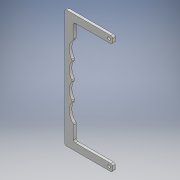
# Autodesk Inventor part: handle_v3
Saved by Autodesk Inventor 2018 (Build 220112000, 112)
## iProperties
Created: 2018-05-21
Part Number: handle_v3
Material: Generic
Document SubType Name: Modeling
Designer: etd
Density: 1 g/cm^3
Appearance: Default
Author: etd
Autodesk Inventor part; units mm, degrees
ref_plane "YZ Plane" through (0, 0, 0) normal (1, 0, 0) x (0, 1, 0)
ref_plane "XZ Plane" through (0, 0, 0) normal (0, 1, 0) x (-1, 0, 0)
ref_plane "XY Plane" through (0, 0, 0) normal (0, 0, 1) x (1, 0, 0)
sketch "Sketch1" plane through (0, 0, 0) normal (0, 1, 0) x (-1, 0, 0)
  line L0 (0, 0) -> (50, 0) construction
  line L1 (0, 0) -> (0, -62.5) construction
  line L2 (0, -62.5) -> (-4, -62.5) construction
  line L3 (40, -58.5) -> (-4, -58.5)
  line L4 (-4, -58.5) -> (-4, -66.5)
  line L5 (-4, -66.5) -> (50, -66.5)
  line L6 (50, -66.5) -> (50, 66.5)
  line L7 (50, 66.5) -> (-4, 66.5)
  line L8 (-4, 66.5) -> (-4, 58.5)
  line L9 (-4, 58.5) -> (40, 58.5)
  line L10 (40, 58.5) -> (40, -58.5)
  point P0 (0, 62.5)
  dimension "d0" = 62.5
  dimension "d1" = 50
  dimension "d2" = 4
  dimension "d3" = 8
  dimension "d4" = 10
  constraints: 22 end point, 5 perpendicular, 4 horizontal, 2 midpoint, 2 vertical, 1 coincident, 1 symmetric about line, 3 other
  measures "d0" distance of L0.start L1.end
  measures "d1" distance of L0.start L0.end
  measures "d2" distance of L1.end L2.end
  measures "d3" distance of L3.end L4.end
  measures "d4" distance between parallel lines of L6 L10
extrude "Plate1" add sketch "Sketch1" along normal blind 3
hole "Hole1" at (0, 0, -62.5) at (0, 0, 62.5) direction (0, 1, 0) diameter 3 end through all
sketch "Sketch2" plane through (0, 3, 0) normal (0, 1, 0) x (1, 0, 0)
  circle A0 centre (0, 62.5) radius 1.5 projected
  circle A1 centre (0, -62.5) radius 1.5 projected
  line L0 (-40, 58.5) -> (-40, -58.5) projected
  line L1 (4, 58.5) -> (-40, 58.5) projected
  line L2 (4, 66.5) -> (4, 58.5) projected
  line L3 (-50, 66.5) -> (4, 66.5) projected
  line L4 (-50, -66.5) -> (-50, 66.5) projected
  line L5 (4, -66.5) -> (-50, -66.5) projected
  line L6 (4, -58.5) -> (4, -66.5) projected
  line L7 (-40, -58.5) -> (4, -58.5) projected
  circle A2 centre (-30, -30) radius 15
  circle A3 centre (-30, -10) radius 15
  circle A4 centre (-30, 10) radius 15
  circle A5 centre (-30, 30) radius 15
  line L8 (-30, 30) -> (-30, -30) construction
  line L9 (-30, 30) -> (-30, 58.5) construction
  line L10 (-30, -30) -> (-30, -58.5) construction
  point P0 (0, 0)
  dimension "d13" = 20
  dimension "d14" = 20
  dimension "d15" = 30
  dimension "d16" = 20
  dimension "d17" = 10
  constraints: 6 end point, 4 centre point, 4 point on line, 3 equal radius, 3 vertical, 1 collinear
  measures "d13" distance of L8.end A3.centre
  measures "d14" distance of A3.centre A4.centre
  measures "d15" diameter of A2
  measures "d16" distance of L8.start A4.centre
  measures "d17" distance between parallel lines of L0 L10
extrude "Extrusion1" cut sketch "Sketch2" against normal through all contours A5 A4 L0 | L0 A4 A5 | A4 A5 L0 | L0 A5 A4 | A5 L0 A3 A4 | A5 A4 A3 L0 | A4 L0 A2 A3 | A3 L0 A4 | A3 A4 L0 | A3 L0 A2 | A2 L0 A3 | A4 A3 A2 L0 | A2 A3 L0 | L0 A3 A2
fillet "Fillet1" radius 2 8 edges at (-50, 1.5, 66.5) (-40, 1.5, 58.5) (4, 1.5, 66.5) (4, 1.5, 58.5) (4, 1.5, -58.5) (4, 1.5, -66.5) (-40, 1.5, -58.5) (-50, 1.5, -66.5)
fillet "Fillet2" radius 2 5 edges at (-40, 1.5, 41.1803) (-41.1803, 1.5, 20) (-41.1803, 1.5, 0) (-41.1803, 1.5, -20) (-40, 1.5, -41.1803)
equation "\"d0\" = 0.5 * holes_spacing"
equation "\"d1\" = handle_height"
equation "\"d2\" = hole_2_border"
equation "\"d3\" = 2 * hole_2_border"
equation "\"d4\" = handle_width"
equation "\"d11\" = Thickness"
equation "\"d13\" = finger_trace_width"
equation "\"d14\" = finger_trace_width"
equation "\"d15\" = finger_trace_diameter"
equation "\"d16\" = finger_trace_width"
equation "\"d5\" = Thickness"
equation "\"hole_2_border\" = 4"
equation "\"BendRadius\" = Thickness"
equation "\"BendReliefWidth\" = Thickness"
equation "\"BendReliefDepth\" = 0.5 * Thickness"
equation "\"CornerReliefSize\" = 4 * Thickness"
equation "\"MinimumRemnant\" = 2 * Thickness"
equation "\"TransitionRadius\" = BendRadius"
equation "\"JacobiRadiusSize\" = BendRadius"
equation "\"GapSize\" = Thickness"
equation "\"handle_height\" = 50"
equation "\"handle_width\" = 10"
equation "\"finger_trace_diameter\" = 30"
equation "\"finger_trace_width\" = 20"
equation "\"holes_spacing\" = 125"
equation "\"Thickness\" = 3"
body "Solid1"
